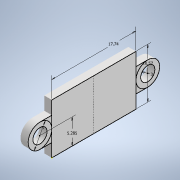
# Autodesk Inventor part: VL53L1X board
Saved by Autodesk Inventor 2022 (Build 260153070, 153G)
## iProperties
Created: 2021-10-27
Part Number: VL53L1X board
Material: Generic
Document SubType Name: Modeling
Designer: a laptop
Density: 1 g/cm^3
Appearance: Default
Author: a laptop
Autodesk Inventor part; units mm, degrees
ref_plane "YZ Plane" through (0, 0, 0) normal (1, 0, 0) x (0, 1, 0)
ref_plane "XZ Plane" through (0, 0, 0) normal (0, 1, 0) x (-1, 0, 0)
ref_plane "XY Plane" through (0, 0, 0) normal (0, 0, 1) x (1, 0, 0)
sketch "Sketch1" plane through (0, 0, 0) normal (1, 0, 0) x (0, 1, 0)
  line L0 (10.57, 0) -> (0, 0)
  line L1 (0, 0) -> (0, -17.74)
  line L2 (0, -17.74) -> (10.57, -17.74)
  line L3 (10.57, -17.74) -> (10.57, 0)
  circle A0 centre (5.285, 2.5) radius 2.5
  circle A1 centre (5.285, 2.5) radius 1.5
  line L4 (10.57, -8.87) -> (0, -8.87) construction
  circle A2 centre (5.285, -20.24) radius 2.5
  circle A3 centre (5.285, -20.24) radius 1.5
  line L5 (7.785, 2.5) -> (7.785, 0)
  line L6 (2.785, 2.5) -> (2.785, 0)
  line L7 (7.785, -20.24) -> (7.785, -17.74)
  line L8 (2.785, -20.24) -> (2.785, -17.74)
  dimension "d0" = 17.74
  dimension "d1" = 10.57
  dimension "d2" = 5.285
  dimension "d3" = 5
  dimension "d11" = 3
  constraints: 18 end point, 5 perpendicular, 5 tangent, 4 centre point, 4 point on circle, 4 point on line, 3 coincident, 2 midpoint, 2 parallel, 2 symmetric about line, 1 horizontal, 2 other
  measures "d0" distance of L2.end L0.start
  measures "d1" distance of L1.end L2.end
  measures "d2" horizontal distance of point (0, 0) A0.centre
  measures "d3" diameter of A0
  measures "d11" diameter of A3
extrude "Extrusion1" add sketch "Sketch1" against normal blind 1.57
body "Solid1"
